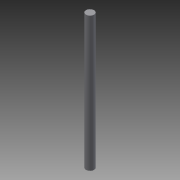
# Autodesk Inventor part: input_spindle
Saved by Autodesk Inventor 2014 (Build 180170000, 170)
## iProperties
Created: 2015-06-18
Part Number: input_spindle
Material: Generic
Document SubType Name: Modeling
Designer: vorac
Density: 1 g/cm^3
Appearance: Default
Author: vorac
Autodesk Inventor part; units mm, degrees
ref_plane "YZ Plane" through (0, 0, 0) normal (1, 0, 0) x (0, 1, 0)
ref_plane "XZ Plane" through (0, 0, 0) normal (0, 1, 0) x (-1, 0, 0)
ref_plane "XY Plane" through (0, 0, 0) normal (0, 0, 1) x (1, 0, 0)
sketch "Sketch1" plane through (0, 0, 0) normal (0, 0, 1) x (1, 0, 0)
  circle A0 centre (0, 0) radius 14.9305
  line L0 (4.7107, 14.1679) -> (-4.7107, 14.1679)
  line L1 (-4.7107, 14.1679) -> (-4.7107, 10.3691)
  line L2 (-4.7107, 10.3691) -> (4.7107, 10.3691)
  line L3 (4.7107, 10.3691) -> (4.7107, 14.1679)
  line L4 (0, 0) -> (0, 27.3143) construction
  point P0 (0, 10.3691)
  dimension "d0" = 29.861
  dimension "d3" = 3.7988
  dimension "d4" = 9.4214
  constraints: 10 end point, 3 perpendicular, 2 point on circle, 1 centre point, 1 coincident, 1 midpoint, 1 point on line, 1 vertical
  measures "d0" diameter of A0
  measures "d3" distance of L2.end L0.start
  measures "d4" distance of L0.start L0.end
extrude "Extrusion1" add sketch "Sketch1" along normal blind 500
body "Solid1"
